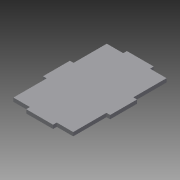
# Autodesk Inventor part: tapadelante
Saved by Autodesk Inventor 2015 (Build 190159000, 159)
## iProperties
Created: 2017-09-28
Part Number: tapadelante
Material: Generic
Document SubType Name: Modeling
Designer: Max
Density: 1 g/cm^3
Appearance: Default
Author: Max
Autodesk Inventor part; units mm, degrees
ref_plane "YZ Plane" through (0, 0, 0) normal (1, 0, 0) x (0, 1, 0)
ref_plane "XZ Plane" through (0, 0, 0) normal (0, 1, 0) x (-1, 0, 0)
ref_plane "XY Plane" through (0, 0, 0) normal (0, 0, 1) x (1, 0, 0)
sketch "Sketch1" plane through (0, 0, 0) normal (0, 0, 1) x (1, 0, 0)
  line L0 (0, 0) -> (89, 0)
  line L1 (89, 0) -> (89, 139)
  line L2 (89, 139) -> (0, 139)
  line L3 (0, 139) -> (0, 0)
  line L4 (24.5, 0) -> (64.5, 0)
  line L5 (64.5, 0) -> (64.5, -5.5)
  line L6 (64.5, -5.5) -> (24.5, -5.5)
  line L7 (24.5, -5.5) -> (24.5, 0)
  line L8 (24.5, 139) -> (64.5, 139)
  line L9 (64.5, 139) -> (64.5, 144.5)
  line L10 (64.5, 144.5) -> (24.5, 144.5)
  line L11 (24.5, 144.5) -> (24.5, 139)
  line L12 (0, 49.5) -> (-5.5, 49.5)
  line L13 (-5.5, 49.5) -> (-5.5, 89.5)
  line L14 (-5.5, 89.5) -> (0, 89.5)
  line L15 (0, 89.5) -> (0, 49.5)
  line L16 (89, 49.5) -> (94.5, 49.5)
  line L17 (94.5, 49.5) -> (94.5, 89.5)
  line L18 (94.5, 89.5) -> (89, 89.5)
  line L19 (89, 89.5) -> (89, 49.5)
  dimension "d5" = 89
  dimension "d6" = 139
  dimension "d7" = 40
  dimension "d8" = 5.5
  dimension "d9" = 40
  dimension "d10" = 5.5
  dimension "d11" = 5.5
  dimension "d12" = 40
  dimension "d13" = 5.5
  dimension "d14" = 40
  constraints: 40 end point, 10 parallel, 5 horizontal, 5 perpendicular, 4 point on line
  measures "d5" distance of L2.end L1.end
  measures "d6" distance of L1.end L0.end
  measures "d7" distance of L5.end L6.end
  measures "d8" distance of L4.end L5.end
  measures "d9" distance of L10.end L9.end
  measures "d10" distance of L9.end L8.end
  measures "d11" distance of L13.end L14.end
  measures "d12" distance of L12.end L13.end
  measures "d13" distance of L18.end L17.end
  measures "d14" distance of L17.end L16.end
extrude "Extrusion1" add sketch "Sketch1" along normal blind 5.5
body "Solid1"
